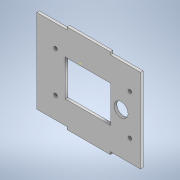
# Autodesk Inventor part: Level2-3 (GLCD)
Saved by Autodesk Inventor 2020 (Build 240168000, 168)
## iProperties
Created: 2020-01-31
Part Number: Level2-3 (GLCD)
Material: Generic
Document SubType Name: Modeling
Designer: jelte
Density: 1 g/cm^3
Appearance: Default
Mass: 28.4701 g
Surface Area: 213.7 cm^2
Volume: 28.4701 cm^3
Author: jelte
Autodesk Inventor part; units mm, degrees
ref_plane "YZ Plane" through (0, 0, 0) normal (1, 0, 0) x (0, 1, 0)
ref_plane "XZ Plane" through (0, 0, 0) normal (0, 1, 0) x (-1, 0, 0)
ref_plane "XY Plane" through (0, 0, 0) normal (0, 0, 1) x (1, 0, 0)
sketch "Sketch2" plane through (0, 0, 0) normal (0, 0, 1) x (1, 0, 0)
  line L0 (-50.1541, 26.4593) -> (-15.1541, 26.4593)
  line L1 (-15.1541, 26.4593) -> (-15.1541, 29.4593)
  line L2 (-15.1541, 29.4593) -> (34.8459, 29.4593)
  line L3 (34.8459, 29.4593) -> (34.8459, 26.4593)
  line L4 (34.8459, 26.4593) -> (69.8459, 26.4593)
  line L5 (-50.1541, 26.4593) -> (-50.1541, -70.5407)
  line L6 (-50.1541, -70.5407) -> (-15.1541, -70.5407)
  line L7 (-15.1541, -70.5407) -> (-15.1541, -73.5407)
  line L8 (-15.1541, -73.5407) -> (34.8459, -73.5407)
  line L9 (34.8459, -73.5407) -> (34.8459, -70.5407)
  line L10 (34.8459, -70.5407) -> (69.8459, -70.5407)
  line L11 (69.8459, -70.5407) -> (69.8459, 26.4593)
  point P0 (0, 0)
  dimension "d0" = 3
  dimension "d1" = 50
  dimension "d2" = 35
  dimension "d3" = 35
  dimension "d4" = 97
  dimension "d5" = 97
  dimension "d6" = 3
  dimension "d7" = 35
  dimension "d8" = 50
  dimension "d9" = 35
  constraints: 24 end point, 7 perpendicular, 4 point on line, 2 horizontal, 1 vertical
  measures "d0" distance of L0.end L1.end
  measures "d1" distance of L1.end L2.end
  measures "d2" distance of L3.end L4.end
  measures "d3" distance of L0.start L0.end
  measures "d4" distance of L0.start L5.end
  measures "d5" distance of L10.end L4.end
  measures "d6" distance of L6.end L7.end
  measures "d7" distance of L5.end L6.end
  measures "d8" distance of L7.end L8.end
  measures "d9" distance of L9.end L10.end
extrude "Extrusion1" add sketch "Sketch2" along normal blind 3
sketch "Sketch3" plane through (0, 0, 3) normal (0, 0, 1) x (1, 0, 0)
  line L0 (34.8459, 29.4593) -> (-15.1541, 29.4593) projected
  line L1 (-15.1541, -73.5407) -> (34.8459, -73.5407) projected
  line L2 (-50.1541, 26.4593) -> (-50.1541, -70.5407) projected
  line L3 (69.8459, -70.5407) -> (69.8459, 26.4593) projected
  circle A0 centre (57.6459, 1.2193) radius 2
  circle A1 centre (57.6459, -45.5807) radius 2
  circle A2 centre (-28.3541, 1.2193) radius 2
  circle A3 centre (-28.3541, -45.5807) radius 2
  circle A4 centre (47.3959, -22.1807) radius 7
  line L4 (-16.4541, -2.7807) -> (34.4459, -2.7807)
  line L5 (34.4459, -2.7807) -> (34.4459, -42.7807)
  line L6 (34.4459, -42.7807) -> (-16.4541, -42.7807)
  line L7 (-16.4541, -42.7807) -> (-16.4541, -2.7807)
  line L8 (-38.3241, -7.0307) -> (-31.4241, -7.0307)
  line L9 (-31.4241, -7.0307) -> (-31.4241, -37.4307)
  line L10 (-31.4241, -37.4307) -> (-38.3241, -37.4307)
  line L11 (-38.3241, -37.4307) -> (-38.3241, -7.0307)
  point P0 (0, 0)
  dimension "d30" = 4
  dimension "d34" = 4
  dimension "d35" = 4
  dimension "d36" = 4
  dimension "d38" = 14
  dimension "d43" = 50.9
  dimension "d44" = 40
  constraints: 16 end point, 5 centre point, 4 parallel, 2 horizontal, 2 perpendicular
  measures "d30" diameter of A1
  measures "d34" diameter of A2
  measures "d35" diameter of A3
  measures "d36" diameter of A0
  measures "d38" diameter of A4
  measures "d43" distance of L4.start L4.end
  measures "d44" distance of L4.end L5.end
extrude "Extrusion2" cut sketch "Sketch3" against normal blind 10
sketch "Sketch4" plane through (-38.3241, -37.4307, 3) normal (1, 0, 0) x (0, 0, -1)
  line L0 (0, 30.4) -> (3, 30.4)
  line L1 (3, 30.4) -> (3, 0)
  line L2 (3, 0) -> (0, 0)
  line L3 (0, 0) -> (0, 30.4)
  point P0 (3, 37.4307)
  constraints: 8 end point, 2 parallel, 1 horizontal, 1 perpendicular
extrude "Extrusion3" add sketch "Sketch4" along normal blind 10
sketch "Sketch5" plane through (0, 0, 3) normal (0, 0, 1) x (1, 0, 0)
  circle A0 centre (47.3959, -22.1807) radius 7 projected
  circle A1 centre (47.3959, -22.1807) radius 8
  line L0 (-16.4541, -2.7807) -> (34.4459, -2.7807) projected
  line L1 (34.4459, -42.7807) -> (-16.4541, -42.7807) projected
  line L2 (35.4459, -43.7807) -> (-17.4541, -43.7807)
  line L3 (-17.4541, -43.7807) -> (-17.4541, -1.7807)
  line L4 (-17.4541, -1.7807) -> (35.4459, -1.7807)
  line L5 (35.4459, -1.7807) -> (35.4459, -43.7807)
  point P0 (0, 0)
  constraints: 8 end point, 2 parallel, 1 centre point, 1 coincident, 1 horizontal, 1 perpendicular
extrude "Extrusion4" cut sketch "Sketch5" against normal blind 10 contours A0 | A1 | L2 L3 L4 L5
sketch "Sketch6" plane through (0, 0, 3) normal (0, 0, 1) x (1, 0, 0)
  point P0 (0, 0)
sketch "Sketch7" plane through (0, 0, 3) normal (0, 0, 1) x (1, 0, 0)
  point P0 (0, 0)
body "Solid1"
